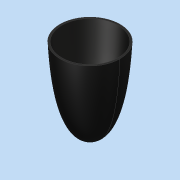
# Autodesk Inventor part: primarySingleFore_02
Saved by Autodesk Inventor 2017 (Build 210142000, 142)
## iProperties
Created: 2016-09-09
Part Number: primarySingleFore_02
Material: Generic
Document SubType Name: Modeling
Designer: techn
Density: 1 g/cm^3
Appearance: Glossy - Black
Mass: 764.223 g
Surface Area: 456.432 cm^2
Volume: 764.223 cm^3
Author: techn
Autodesk Inventor part; units mm, degrees
ref_plane "YZ Plane" through (0, 0, 0) normal (1, 0, 0) x (0, 1, 0)
ref_plane "XZ Plane" through (0, 0, 0) normal (0, 1, 0) x (-1, 0, 0)
ref_plane "XY Plane" through (0, 0, 0) normal (0, 0, 1) x (1, 0, 0)
sketch "Sketch6" plane through (0, 0, 0) normal (0, 0, 1) x (1, 0, 0)
  line L0 (540.6478, 1219.1491) -> (540.6478, -58.7076) construction
  line L1 (540.6478, -58.7076) -> (-407.4394, -58.7076) construction
  line L2 (-407.4394, -58.7076) -> (-407.4394, 1219.1491) construction
  line L3 (-407.4394, 1219.1491) -> (540.6478, 1219.1491) construction
  point P0 (0, 0)
  constraints: 2 other
sketch "Sketch5" plane through (0, 0, 0) normal (0, 0, 1) x (1, 0, 0)
  line L0 (0, 0) -> (0, 142.24)
  line L1 (0, 142.24) -> (50.8, 142.24)
  line L2 (50.8, 142.24) -> (-50.8, 142.24)
  line L3 (50.8, 142.24) -> (43.834, 0) construction
  line L4 (43.834, 0) -> (0, 0) construction
  spline S0 degree 2 poles (50.8, 142.24) (43.834, 0) (0, 0) knots 1 1 1 2 2 2
  line L5 (-50.8, 142.24) -> (-43.834, 0) construction
  line L6 (-43.834, 0) -> (0, 0) construction
  spline S1 degree 2 poles (-50.8, 142.24) (-43.834, 0) (0, 0) knots 1 1 1 2 2 2
  dimension "d20" = 142.24
  dimension "d21" = 50.8
  dimension "d22" = 101.6
  constraints: 6 end point, 1 horizontal, 1 perpendicular, 1 point on line, 1 symmetric about line, 1 vertical, 6 other
  measures "d20" distance of L0.start L0.end
  measures "d21" distance of L0.end L1.end
  measures "d22" distance of L1.end L2.end
revolve "Revolution1" add sketch "Sketch5" angle 360 about axis through (0, 0, 0) along (0, 1, 0) contours L0 L1 S0
shell "Shell1" thickness 3.175 removed faces 1 at (-7.3018, 142.24, -11.5135)
body "Solid1"
